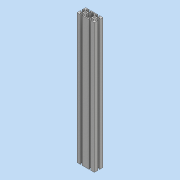
# Autodesk Inventor part: Profil aluminiowy alutec K&K 104080
Saved by Autodesk Inventor 2018 (Build 220112000, 112)
## iProperties
Created: 2019-01-26
Part Number: Profil aluminiowy alutec K&K 104080
Material: Ogólny
Document SubType Name: Modeling
Designer: Dawid
Density: 1 g/cm^3
Appearance: Aluminium odlewane
Author: Dawid
Autodesk Inventor part; units mm, degrees
ref_plane "YZ Plane" through (0, 0, 0) normal (1, 0, 0) x (0, 1, 0)
ref_plane "XZ Plane" through (0, 0, 0) normal (0, 1, 0) x (-1, 0, 0)
ref_plane "XY Plane" through (0, 0, 0) normal (0, 0, 1) x (1, 0, 0)
sketch "Szkic1" plane through (0, 0, 0) normal (0, 0, 1) x (1, 0, 0)
  line L0 (-40, -20.0066) -> (-24.1053, -20.0066)
  circle A0 centre (-20.0066, 0.0296) radius 3.6988
  line L1 (-24.1053, 19.9934) -> (-24.1053, 16.0243)
  line L2 (-15.8947, 19.9934) -> (-15.8947, 15.9947)
  line L3 (-40, -4.0986) -> (-35.9881, -4.0986)
  line L4 (-40, 4.1282) -> (-36.0013, 4.1282)
  line L5 (-24.1053, -20.0066) -> (-24.1053, -15.9947)
  line L6 (-15.8947, -20.0066) -> (-15.8947, -16.0079)
  line L7 (-36.0013, 10.0263) -> (-36.0013, 4.1282)
  line L8 (-35.9881, -4.0986) -> (-35.9881, -9.9967)
  line L9 (-24.1053, 16.0243) -> (-30.0033, 16.0243)
  line L10 (-24.1053, 19.9934) -> (-40, 19.9934)
  line L11 (-29.9901, -15.9947) -> (-24.1053, -15.9947)
  line L12 (-40, -20.0066) -> (-24.1053, -20.0066)
  line L13 (-27.7041, 0.0296) -> (-27.7041, 4.8995)
  line L14 (-24.8766, 7.727) -> (-20.0066, 7.727)
  line L15 (-15.0939, 7.727) -> (-20.0066, 7.727)
  line L16 (-12.2664, 4.8995) -> (-12.2664, 0.0296)
  line L17 (-12.2664, 0.0296) -> (-12.2664, -4.8832)
  line L18 (-19.9771, -7.7107) -> (-15.0939, -7.7107)
  line L19 (-19.9771, -7.7107) -> (-24.8338, -7.7107)
  line L20 (-27.7041, -4.8404) -> (-27.7041, 0.0296)
  line L21 (-30.0033, 12.8537) -> (-24.8766, 7.727)
  line L22 (-32.8308, 10.0263) -> (-27.7041, 4.8995)
  line L23 (-30.0033, 16.0243) -> (-30.0033, 12.8537)
  line L24 (-36.0013, 10.0263) -> (-32.8308, 10.0263)
  line L25 (-32.8339, -9.9967) -> (-27.7041, -4.8404)
  line L26 (-29.9901, -12.8405) -> (-24.8338, -7.7107)
  line L27 (-29.9901, -12.8405) -> (-30.0033, -12.8536)
  line L28 (-30.0033, -15.9947) -> (-29.9901, -15.9947)
  line L29 (-29.9901, -15.9947) -> (-29.9901, -12.8405)
  line L30 (-35.9881, -9.9967) -> (-32.8339, -9.9967)
  line L31 (-7.883, 9.2829) -> (-5.998, 11.1679)
  line L32 (-7.883, 9.2829) -> (-12.2664, 4.8995)
  line L33 (-10.7105, 12.1104) -> (-9.9967, 12.8242)
  line L34 (-10.7105, 12.1104) -> (-15.0939, 7.727)
  line L35 (-40, 19.9934) -> (-40, 19.9934)
  line L36 (-9.9967, 15.9947) -> (-9.9967, 12.8242)
  line L37 (0, 15.9947) -> (-1.1712, 15.9947)
  line L38 (-9.9967, 15.9947) -> (-15.8947, 15.9947)
  line L39 (-7.2141, -9.9355) -> (-5.9817, -11.1679)
  line L40 (-7.2141, -9.9355) -> (-12.2664, -4.8832)
  line L41 (-3.9823, -15.9947) -> (-5.9817, -15.9947)
  line L42 (-9.9804, -16.0079) -> (-9.9804, -12.8374)
  line L43 (-5.998, 15.9947) -> (-5.998, 11.1679)
  line L44 (-1.1712, 15.9947) -> (-5.998, 15.9947)
  line L45 (-9.9967, 15.9947) -> (-9.9804, 15.9947)
  line L46 (-5.998, -15.9947) -> (-5.9817, -15.9947)
  line L47 (-5.9817, -15.9947) -> (-5.9817, -11.1679)
  line L48 (-15.8947, -16.0079) -> (-9.9804, -16.0079)
  line L49 (-5.9817, -15.9947) -> (0, -15.9947)
  circle A1 centre (20.0066, 0.0296) radius 3.6988
  line L50 (24.1053, 19.9934) -> (24.1053, 16.0243)
  line L51 (15.9101, 19.9934) -> (15.9101, 15.9947)
  line L52 (40, -4.0986) -> (35.9881, -4.0986)
  line L53 (40, 4.1282) -> (36.0013, 4.1282)
  line L54 (24.1206, -20.0066) -> (24.1206, -15.95)
  line L55 (15.8947, -20.0066) -> (15.8947, -16.0079)
  line L56 (36.0013, 10.0263) -> (36.0013, 4.1282)
  line L57 (35.9881, -4.0986) -> (35.9881, -9.9967)
  line L58 (24.1053, 16.0243) -> (30.0186, 16.0243)
  line L59 (24.1053, 19.9934) -> (40, 19.9934)
  line L60 (30.0054, -15.95) -> (24.1206, -15.95)
  line L61 (27.7041, 0.0296) -> (27.7041, 4.8995)
  line L62 (24.8919, 7.7717) -> (20.0219, 7.7717)
  line L63 (15.1092, 7.7717) -> (20.0219, 7.7717)
  line L64 (12.2664, 4.8995) -> (12.2664, 0.0296)
  line L65 (12.2664, 0.0296) -> (12.2664, -4.8832)
  line L66 (27.7041, -4.8404) -> (27.7041, 0.0296)
  line L67 (30.0186, 12.8985) -> (24.8919, 7.7717)
  line L68 (32.8308, 10.0263) -> (27.7041, 4.8995)
  line L69 (30.0186, 16.0243) -> (30.0186, 12.8985)
  line L70 (36.0013, 10.0263) -> (32.8308, 10.0263)
  line L71 (32.8339, -9.9967) -> (27.7041, -4.8404)
  line L72 (30.0186, -15.95) -> (30.0054, -15.95)
  line L73 (35.9881, -9.9967) -> (32.8339, -9.9967)
  line L74 (7.883, 9.2829) -> (5.998, 11.1679)
  line L75 (7.883, 9.2829) -> (12.2664, 4.8995)
  line L76 (10.7258, 12.1551) -> (10.012, 12.8689)
  line L77 (10.7258, 12.1551) -> (15.1092, 7.7717)
  line L78 (40, 19.9934) -> (40, 19.9934)
  line L79 (10.012, 15.9947) -> (10.012, 12.8689)
  line L80 (0, 15.9947) -> (1.1712, 15.9947)
  line L81 (10.012, 15.9947) -> (15.9101, 15.9947)
  line L82 (7.2141, -9.9355) -> (5.9817, -11.1679)
  line L83 (7.2141, -9.9355) -> (12.2664, -4.8832)
  line L84 (10.0416, -12.7762) -> (15.0939, -7.7239)
  line L85 (3.9823, -15.9947) -> (5.9817, -15.9947)
  line L86 (9.9804, -16.0079) -> (9.9804, -12.8374)
  line L87 (10.0416, -12.7762) -> (9.9804, -12.8374)
  line L88 (5.998, 15.9947) -> (5.998, 11.1679)
  line L89 (1.1712, 15.9947) -> (5.998, 15.9947)
  line L90 (10.012, 15.9947) -> (9.9804, 15.9947)
  line L91 (5.998, -15.9947) -> (5.9817, -15.9947)
  line L92 (5.9817, -15.9947) -> (5.9817, -11.1679)
  line L93 (15.8947, -16.0079) -> (9.9804, -16.0079)
  line L94 (5.9817, -15.9947) -> (0, -15.9947)
  line L95 (0, 16.0243) -> (0, 15.9947)
  line L96 (0, -20.0066) -> (0, -19.9934)
  line L97 (0, -16.0079) -> (0, -15.9947)
  line L98 (-40, 4.1282) -> (-40, 19.9934)
  line L99 (-40, -4.0986) -> (-40, -20.0066)
  line L100 (40, 4.1282) -> (40, 19.9934)
  line L101 (40, -20.0066) -> (40, -4.0986)
  line L102 (24.1206, -20.0066) -> (40, -20.0066)
  line L103 (24.8766, -7.7239) -> (15.0939, -7.7239)
  line L104 (30.0186, -15.95) -> (30.0186, -12.8089)
  line L105 (30.0186, -12.8089) -> (24.8766, -7.7239)
  line L106 (-15.8947, -20.0066) -> (15.8947, -20.0066)
  line L107 (-9.9804, -12.8374) -> (-15.0939, -7.7107)
  line L108 (-15.8947, 19.9934) -> (15.9101, 19.9934)
  point P0 (0, 0)
  dimension "d54" = 40
  dimension "d56" = 80
  dimension "d57" = 80
  dimension "d61" = 40
  dimension "d62" = 40
  dimension "d65" = 0
  dimension "d66" = 0
  constraints: 218 end point, 17 perpendicular, 17 point on line, 9 horizontal, 6 vertical, 2 centre point, 2 parallel, 1 collinear
  measures "d54" distance between parallel lines of L0 L10
  measures "d56" distance between parallel lines of L100 L98
  measures "d57" distance between parallel lines of L101 L99
  measures "d61" distance between parallel lines of L102 L59
  measures "d62" distance between parallel lines of L106 L108
  measures "d65" distance between parallel lines of L10 L108
  measures "d66" distance between parallel lines of L59 L108
extrude "Wyciągnięcie proste2" add sketch "Szkic1" along normal blind 600
